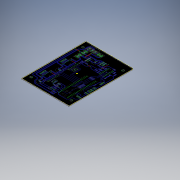
# Autodesk Inventor part: PCB
Saved by Autodesk Inventor 2019 (Build 230136000, 136)
## iProperties
Created: 2021-11-23
Part Number: PCB
Material: Generic
Document SubType Name: Modeling
Designer: Pokick
Density: 1 g/cm^3
Appearance: Default
Author: Pokick
Autodesk Inventor part; units mm, degrees
ref_plane "YZ Plane" through (0, 0, 0) normal (1, 0, 0) x (0, 1, 0)
ref_plane "XZ Plane" through (0, 0, 0) normal (0, 1, 0) x (-1, 0, 0)
ref_plane "XY Plane" through (0, 0, 0) normal (0, 0, 1) x (1, 0, 0)
sketch "Sketch1" plane through (0, 0, 0) normal (0, 1, 0) x (-1, 0, 0)
  line L0 (-35, 45) -> (35, 45) construction
  line L1 (35, 45) -> (35, -45) construction
  line L2 (35, -45) -> (-35, -45) construction
  line L3 (-35, -45) -> (-35, 45) construction
  line L4 (-35, 45) -> (35, -45) construction
  line L5 (35, 45) -> (-35, -45) construction
  line L6 (-41, -55) -> (41, -55)
  line L7 (41, -55) -> (41, 55)
  line L8 (41, 55) -> (-41, 55)
  line L9 (-41, 55) -> (-41, -55)
  line L10 (-41, -55) -> (41, 55) construction
  line L11 (41, -55) -> (-41, 55) construction
  circle A0 centre (35, 45) radius 1.6
  circle A1 centre (35, -45) radius 1.6
  circle A2 centre (-35, -45) radius 1.6
  circle A3 centre (-35, 45) radius 1.6
  point P0 (0, 0)
  dimension "d0" = 70
  dimension "d1" = 90
  dimension "d2" = 82
  dimension "d3" = 110
  dimension "d4" = 3.2
  dimension "d5" = 3.2
  dimension "d6" = 3.2
  dimension "d7" = 3.2
  constraints: 24 end point, 4 centre point, 4 coincident, 4 midpoint, 4 parallel, 2 horizontal, 2 perpendicular
  measures "d0" distance of L1.end L2.end
  measures "d1" distance of L0.end L1.end
  measures "d2" distance of L8.end L7.end
  measures "d3" distance of L7.end L6.end
  measures "d4" diameter of A0
  measures "d5" diameter of A1
  measures "d6" diameter of A2
  measures "d7" diameter of A3
extrude "Extrusion1" add sketch "Sketch1" along normal blind 1
sketch "Sketch2" plane through (0, 1, 0) normal (0, 1, 0) x (1, 0, 0)
  line L0 (-40.4315, -54.7325) -> (-40.4315, 56.2757) construction
  line L1 (-40.4315, 56.2757) -> (41.3362, 56.2757) construction
  line L2 (41.3362, 56.2757) -> (41.3362, -54.7325) construction
  line L3 (41.3362, -54.7325) -> (-40.4315, -54.7325) construction
  point P0 (0, 0)
  constraints: 2 other
body "Solid1"
